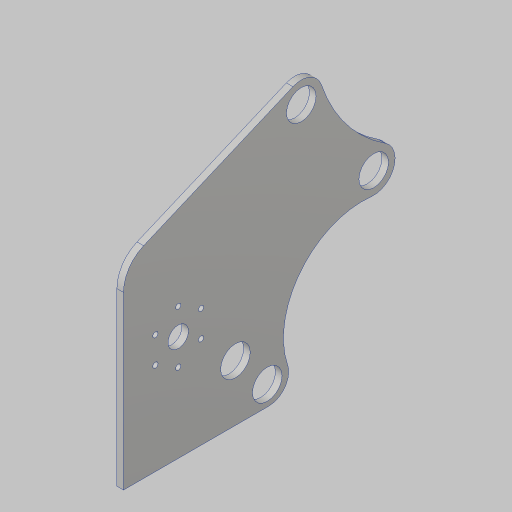
# Autodesk Inventor part: GI - 001
Saved by Autodesk Inventor 2023.5 (Build 275446000, 446)
## iProperties
Created: 2025-01-17
Part Number: GI - 001
Material: Aluminum 6061
Document SubType Name: Modeling
Designer: mavericks
Density: 2.7 g/cm^3
Appearance: Aluminum - Flat
Author: mavericks
Autodesk Inventor part; units mm, degrees
ref_plane "YZ Plane" through (0, 0, 0) normal (1, 0, 0) x (0, 1, 0)
ref_plane "XZ Plane" through (0, 0, 0) normal (0, 1, 0) x (-1, 0, 0)
ref_plane "XY Plane" through (0, 0, 0) normal (0, 0, 1) x (1, 0, 0)
sketch "Sketch2" plane through (0, 0, 0) normal (1, 0, 0) x (0, 1, 0)
  line L0 (63.5, 38.1) -> (-63.5, 38.1) construction
  line L1 (-63.5, 38.1) -> (-63.5, -38.1) construction
  line L2 (-63.5, -38.1) -> (63.5, -38.1) construction
  line L3 (63.5, -38.1) -> (63.5, 38.1) construction
  line L4 (63.5, 38.1) -> (-63.5, -38.1) construction
  line L5 (-63.5, 38.1) -> (63.5, -38.1) construction
  line L6 (-63.5, 38.1) -> (-76.2, 38.1) construction
  line L7 (-76.2, 38.1) -> (-76.2, -266.7) construction
  line L8 (-76.2, -266.7) -> (-63.5, -266.7) construction
  line L9 (-63.5, -266.7) -> (-63.5, 38.1) construction
  circle A0 centre (4.5591, -357.9215) radius 57.15 construction
  circle A1 centre (-50.8, -100.5497) radius 15.875 construction
  circle A2 centre (-15.875, -69.85) radius 25.4 construction
  circle A3 centre (76.2, -203.2) radius 63.5 construction
  circle A4 centre (76.2, -203.2) radius 14.2875
  circle A5 centre (166.2946, -133.35) radius 38.1 construction
  circle A6 centre (166.2946, -133.35) radius 14.2875
  circle A7 centre (-50.8, -100.5497) radius 14.2875
  circle A8 centre (-15.875, -69.85) radius 14.2875
  line L10 (-69.85, 38.1) -> (-69.85, -102.1372)
  arc A9 (-50.8, -121.1872) -> (-44.2424, -120.1177) centre (-50.8, -100.5497) ccw
  arc A10 (55.692, -200.8917) -> (93.5118, -214.4342) centre (76.2, -203.2) ccw
  arc A11 (172.8612, -152.9149) -> (185.307, -125.3228) centre (166.2946, -133.35) ccw
  arc A12 (55.692, -200.8917) -> (-44.2424, -120.1177) centre (-20.0298, -192.3686) ccw
  line L11 (-69.85, 38.1) -> (95.25, 38.1)
  line L12 (124.4998, 18.6995) -> (185.307, -125.3228)
  arc A13 (172.8612, -152.9149) -> (93.5118, -214.4342) centre (221.353, -297.3944) ccw
  arc A14 (124.4998, 18.6995) -> (95.25, 38.1) centre (95.25, 6.35) ccw
  arc A15 (-69.85, -102.1372) -> (-50.8, -121.1872) centre (-50.8, -102.1372) ccw
  line L13 (-57.15, 38.1) -> (-6.35, 38.1) construction
  line L14 (-6.35, 38.1) -> (-6.35, 444.5) construction
  line L15 (-6.35, 444.5) -> (-57.15, 444.5) construction
  line L16 (-57.15, 444.5) -> (-57.15, 38.1) construction
  point P0 (0, 0)
  point P1 (-14.3002, 165.1)
  point P2 (-49.1998, 165.1)
  point P3 (-14.3002, 190.5)
  point P4 (-49.1998, 190.5)
  point P5 (-14.3002, 215.9)
  point P6 (-49.1998, 215.9)
  point P7 (-14.3002, 241.3)
  point P8 (-49.1998, 241.3)
  dimension "d2" = 127
  dimension "d3" = 76.2
  dimension "d4" = 12.7
  dimension "d5" = 304.8
  dimension "d6" = 114.3
  dimension "d7" = 31.75
  dimension "d8" = 50.8
  dimension "d9" = 127
  dimension "d10" = 152.4
  dimension "d11" = 28.575
  dimension "d12" = 31.75
  dimension "d13" = 25.4
  dimension "d14" = 46.4998
  dimension "d15" = 47.625
  dimension "d16" = 165.1
  dimension "d17" = 76.2
  dimension "d18" = 114.0003
  dimension "d19" = 69.85
  dimension "d20" = 28.575
  dimension "d21" = 28.575
  dimension "d22" = 28.575
  dimension "d23" = 6.35
  dimension "d24" = 6.35
  dimension "d25" = 6.35
  dimension "d26" = 76.2
  dimension "d28" = 165.1
  dimension "d29" = 152.4
  dimension "d30" = 31.75
  dimension "d35" = 19.05
  dimension "d40" = 50.8
  dimension "d41" = 19.05
  dimension "d42" = 406.4
  dimension "d43" = 127
  dimension "d44" = 7.9502
  dimension "d45" = 7.9502
  dimension "d48" = 25.4
  constraints: 34 end point, 16 centre point, 14 point on circle, 10 tangent, 6 parallel, 4 coincident, 4 perpendicular, 3 horizontal, 3 midpoint, 1 horizontal alignment, 1 point on line, 1 vertical, 6 other
  measures "d2" distance of L2.end L1.end
  measures "d3" distance of L1.end L0.end
  measures "d4" distance of L8.end L7.end
  measures "d5" distance of L7.end L6.end
  measures "d6" diameter of A0
  measures "d7" diameter of A1
  measures "d8" diameter of A2
  measures "d9" diameter of A3
  measures "d10" distance from line of A3.centre L7
  measures "d11" diameter of A4
  measures "d12" distance from line of A2.centre L2
  measures "d13" distance from line of L7 A1.centre
  measures "d14" distance of A2.centre A1.centre
  measures "d15" distance from line of L9 A2.centre
  measures "d16" distance from line of L2 A3.centre
  measures "d17" diameter of A5
  measures "d18" distance of A3.centre A5.centre
  measures "d19" vertical distance of A5.centre A3.centre
  measures "d20" diameter of A6
  measures "d21" diameter of A7
  measures "d22" diameter of A8
  measures "d23" radial gap between concentric circles of A7 A9
  measures "d24" radial gap between concentric circles of A4 A10
  measures "d25" radial gap between concentric circles of A6 A11
  measures "d26" radius of A12
  measures "d28" distance of L11.end L10.start
  measures "d29" radius of A13
  measures "d30" radius of A14
  measures "d35" radius of A15
  measures "d40" distance of L15.end L14.end
  measures "d41" distance between parallel lines of L16 L7
  measures "d42" distance of L15.end L13.start
  measures "d43" distance from line of L0 point (-14.3, 165.1)
  measures "d44" distance from line of L14 point (-14.3, 165.1)
  measures "d45" distance from line of L16 point (-49.2, 165.1)
  measures "d48" distance of point (-14.3, 165.1) point (-14.3, 190.5)
extrude "Extrusion1" add sketch "Sketch2" along normal blind 6.35
sketch "Sketch3" plane through (6.35, 0, 0) normal (1, 0, 0) x (0, 0, -1)
  line L0 (-38.1, 63.5) -> (38.1, 63.5) construction
  line L1 (38.1, 63.5) -> (38.1, -63.5) construction
  line L2 (38.1, -63.5) -> (-38.1, -63.5) construction
  line L3 (-38.1, -63.5) -> (-38.1, 63.5) construction
  line L4 (-38.1, 63.5) -> (38.1, -63.5) construction
  line L5 (38.1, 63.5) -> (-38.1, -63.5) construction
  line L6 (-38.1, -69.85) -> (102.1372, -69.85) construction
  line L7 (-38.1, 95.25) -> (-38.1, -69.85) construction
  point P0 (0, 0)
  point P1 (0, 0)
  dimension "d36" = 76.2
  dimension "d37" = 127
  dimension "d38" = 6.35
  dimension "d39" = 0
  constraints: 12 end point, 2 midpoint, 2 parallel, 1 horizontal, 1 perpendicular
  measures "d36" distance of L1.end L2.end
  measures "d37" distance of L0.end L1.end
  measures "d38" distance between parallel lines of L6 L2
  measures "d39" distance between parallel lines of L7 L3
sketch "Sketch4" plane through (0, 0, 0) normal (-1, 0, 0) x (0, 0, 1)
  circle A0 centre (-14.6898, 31.75) radius 9.906
  circle A1 centre (-203.2, 76.2) radius 14.2875 projected
  circle A2 centre (-133.35, 166.2946) radius 14.2875 projected
  circle A3 centre (-100.5497, -50.8) radius 14.2875 projected
  circle A4 centre (-69.85, -15.875) radius 14.2875 projected
  arc A5 (38.1, 95.25) -> (18.6995, 124.4998) centre (6.35, 95.25) ccw projected
  line L0 (38.1, 95.25) -> (38.1, -69.85) projected
  line L1 (38.1, -69.85) -> (-102.1372, -69.85) projected
  arc A6 (-121.1872, -50.8) -> (-102.1372, -69.85) centre (-102.1372, -50.8) ccw projected
  arc A7 (-120.1177, -44.2424) -> (-121.1872, -50.8) centre (-100.5497, -50.8) ccw projected
  arc A8 (-120.1177, -44.2424) -> (-200.8917, 55.692) centre (-192.3686, -20.0298) ccw projected
  arc A9 (-214.4342, 93.5118) -> (-200.8917, 55.692) centre (-203.2, 76.2) ccw projected
  arc A10 (-214.4342, 93.5118) -> (-152.9149, 172.8612) centre (-297.3944, 221.353) ccw projected
  arc A11 (-125.3228, 185.307) -> (-152.9149, 172.8612) centre (-133.35, 166.2946) ccw projected
  line L2 (-125.3228, 185.307) -> (18.6995, 124.4998) projected
  circle A12 centre (-203.2, 76.2) radius 14.2875 projected
  circle A13 centre (-133.35, 166.2946) radius 14.2875 projected
  circle A14 centre (-100.5497, -50.8) radius 14.2875 projected
  circle A15 centre (-69.85, -15.875) radius 14.2875 projected
  arc A16 (38.1, 95.25) -> (18.6995, 124.4998) centre (6.35, 95.25) ccw projected
  line L3 (38.1, 95.25) -> (38.1, -69.85) projected
  line L4 (38.1, -69.85) -> (-102.1372, -69.85) projected
  arc A17 (-121.1872, -50.8) -> (-102.1372, -69.85) centre (-102.1372, -50.8) ccw projected
  arc A18 (-120.1177, -44.2424) -> (-121.1872, -50.8) centre (-100.5497, -50.8) ccw projected
  arc A19 (-120.1177, -44.2424) -> (-200.8917, 55.692) centre (-192.3686, -20.0298) ccw projected
  arc A20 (-214.4342, 93.5118) -> (-200.8917, 55.692) centre (-203.2, 76.2) ccw projected
  arc A21 (-214.4342, 93.5118) -> (-152.9149, 172.8612) centre (-297.3944, 221.353) ccw projected
  arc A22 (-125.3228, 185.307) -> (-152.9149, 172.8612) centre (-133.35, 166.2946) ccw projected
  line L5 (-125.3228, 185.307) -> (18.6995, 124.4998) projected
  circle A23 centre (-14.6898, 31.75) radius 25.4 construction
  point P0 (0, 0)
  point P1 (-14.6898, 57.15)
  point P2 (-36.6869, 44.45)
  point P3 (-36.6869, 19.05)
  point P4 (-14.6898, 6.35)
  point P5 (7.3072, 19.05)
  point P6 (7.3072, 44.45)
  dimension "d58" = 50.8
  dimension "d53" = 19.812
  dimension "d54" = 72.8751
  dimension "d55" = 101.6
  dimension "d61" = 360
  constraints: 2 vertical alignment, 1 centre point, 1 coincident, 9 other
  measures "d53" diameter of A0
  measures "d54" distance of A0.centre A4.centre
  measures "d55" distance from line of L1 A0.centre
extrude "Extrusion2" cut sketch "Sketch4" against normal blind 25.4 contours A0
hole "Hole1" at (0, 57.15, -14.6898) at (0, 44.45, -36.6869) at (0, 19.05, -36.6869) at (0, 6.35, -14.6898) at (0, 19.05, 7.3072) at (0, 44.45, 7.3072) direction (1, 0, 0) diameter 5.1054 end through all clearance for "Flat Head Machine Screw (82)" size "#10" standard "Ansi Unified Screw Threads"
body "Solid1"
